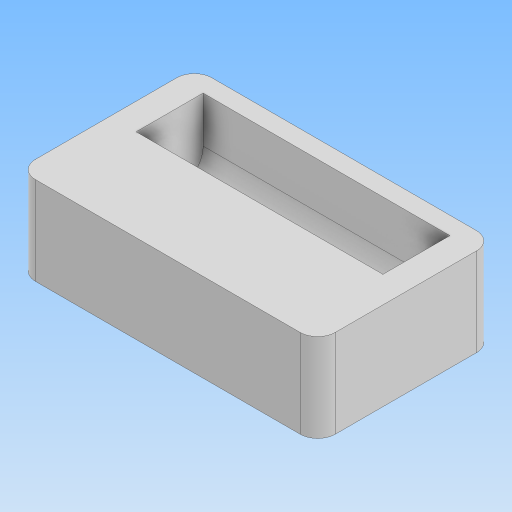
# Autodesk Inventor part: Web_server_holder
Saved by Autodesk Inventor 2024 (Build 280153000, 153)
## iProperties
Created: 2024-02-28
Part Number: Web_server_holder
Material: Generic
Document SubType Name: Modeling
Designer: MenMe
Density: 1 g/cm^3
Appearance: Default
Author: MenMe
Autodesk Inventor part; units mm, degrees
ref_plane "YZ Plane" through (0, 0, 0) normal (1, 0, 0) x (0, 1, 0)
ref_plane "XZ Plane" through (0, 0, 0) normal (0, 1, 0) x (-1, 0, 0)
ref_plane "XY Plane" through (0, 0, 0) normal (0, 0, 1) x (1, 0, 0)
sketch "Sketch1" plane through (0, 0, 0) normal (0, 1, 0) x (-1, 0, 0)
  line L0 (0, 0) -> (85, 0)
  line L1 (85, 0) -> (85, -50)
  line L2 (85, -50) -> (0, -50)
  line L3 (0, -50) -> (0, 0)
  dimension "d0" = 85
  dimension "d1" = 50
  constraints: 8 end point, 2 parallel, 1 horizontal, 1 perpendicular
  measures "d0" distance of L1.end L2.end
  measures "d1" distance of L0.end L1.end
extrude "Extrusion1" add sketch "Sketch1" along normal blind 25
sketch "Sketch2" plane through (0, 25, 0) normal (0, 1, 0) x (1, 0, 0)
  line L0 (-77.5, 26) -> (-7.5, 26)
  line L1 (-7.5, 26) -> (-7.5, 45)
  line L2 (-7.5, 45) -> (-77.5, 45)
  line L3 (-77.5, 45) -> (-77.5, 26)
  line L4 (-85, 50) -> (-85, 0) projected
  line L5 (0, 50) -> (-85, 50) projected
  point P0 (0, 0)
  dimension "d4" = 70
  dimension "d5" = 7.5
  dimension "d6" = 5
  dimension "d7" = 19
  constraints: 8 end point, 2 parallel, 1 horizontal, 1 perpendicular
  measures "d4" distance of L1.end L2.end
  measures "d5" distance between parallel lines of L4 L3
  measures "d6" distance between parallel lines of L5 L2
  measures "d7" distance of L2.end L0.start
extrude "Extrusion2" cut sketch "Sketch2" against normal blind 20
fillet "Fillet1" radius 5 4 edges at (-85, 12.5, 0) (-85, 12.5, -50) (0, 12.5, -50) (0, 12.5, 0)
fillet "Fillet2" radius 7 2 edges at (-42.5, 5, -26) (-42.5, 5, -45)
body "Solid1"
